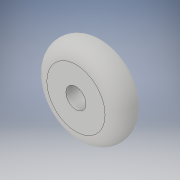
# Autodesk Inventor part: wheel3standin
Saved by Autodesk Inventor 2019 (Build 230136000, 136)
## iProperties
Created: 2019-05-08
Part Number: wheel3standin
Material: Generic
Document SubType Name: Modeling
Designer: Alex Jones
Density: 1 g/cm^3
Appearance: Default
Author: Alex Jones
Autodesk Inventor part; units mm, degrees
ref_plane "YZ Plane" through (0, 0, 0) normal (1, 0, 0) x (0, 1, 0)
ref_plane "XZ Plane" through (0, 0, 0) normal (0, 1, 0) x (-1, 0, 0)
ref_plane "XY Plane" through (0, 0, 0) normal (0, 0, 1) x (1, 0, 0)
sketch "Sketch1" plane through (0, 0, 0) normal (0, 1, 0) x (-1, 0, 0)
  line L0 (-10.75, -3.5) -> (10.75, 3.5) construction
  line L1 (10.75, -3.5) -> (-10.75, 3.5) construction
  line L2 (2.5, 3.5) -> (2.5, -3.5)
  line L3 (-2.5, 3.5) -> (2.5, -3.5) construction
  line L4 (2.5, 3.5) -> (-2.5, -3.5) construction
  arc A0 (7.25, -3.5) -> (7.25, 3.5) centre (7.25, 0) ccw
  line L5 (0, 3.5) -> (0, -3.5)
  line L6 (7.25, -3.5) -> (2.5, -3.5)
  line L7 (2.5, -3.5) -> (2.5, 3.5)
  line L8 (2.5, 3.5) -> (7.25, 3.5)
  line L9 (7.25, 3.5) -> (7.25, -3.5)
  point P0 (0, 0)
  dimension "d0" = 21.5
  constraints: 20 end point, 5 midpoint, 2 parallel, 2 point on circle, 1 centre point, 1 horizontal, 1 perpendicular
  measures "d0" distance of L0.end L1.end
revolve "Revolution1" add sketch "Sketch1" angle 360 about axis through (0, 0, 3.5) along (0, 0, -1)
body "Solid1"
